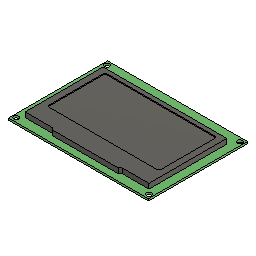
2719 OLED 2.4in (Autodesk Fusion 360 design; units mm, degrees)
Autodesk Fusion 360 part; units mm, degrees
sketch "pcb" plane through (0, 0, 0) normal (0, 0, 1) x (1, 0, 0)
  line L0 (-35, 24.8) -> (35, 24.8)
  line L1 (35, 24.8) -> (35, -24.8)
  line L2 (35, -24.8) -> (-35, -24.8)
  line L3 (-35, -24.8) -> (-35, 24.8)
  line L4 (0, 24.8) -> (0, 0) construction
  line L5 (0, 0) -> (-35, 0) construction
  dimension "d1" = 70
  dimension "d2" = 49.6
  constraint horizontal L0
  constraint vertical L1
  constraint horizontal L2
  constraint vertical L3
  constraint midpoint L0 L4.start
  constraint perpendicular L0 L4
  constraint perpendicular L4 L5
  constraint coincident L4.end L5.start
  constraint midpoint L3 L5.end
  measures "d1" distance of L0.start L0.end
  measures "d2" distance of L0.start L2.end
sketch "holes" plane through (0, 0, 0) normal (0, 0, 1) x (1, 0, 0)
  line L0 (-33.25, 22.75) -> (33.25, 22.75) construction
  line L1 (33.25, 22.75) -> (33.25, -22.75) construction
  line L2 (33.25, -22.75) -> (-33.25, -22.75) construction
  line L3 (-33.25, -22.75) -> (-33.25, 22.75) construction
  line L4 (0, 22.75) -> (0, 0) construction
  line L5 (0, 0) -> (-33.25, 0) construction
  circle A0 centre (-33.25, 22.75) radius 1.25
  circle A1 centre (33.25, 22.75) radius 1.25
  circle A2 centre (33.25, -22.75) radius 1.25
  circle A3 centre (-33.25, -22.75) radius 1.25
  dimension "d3" = 66.5
  dimension "d4" = 45.5
  dimension "d5" = 2.5
  constraint horizontal L0
  constraint vertical L1
  constraint horizontal L2
  constraint vertical L3
  constraint midpoint L0 L4.start
  constraint perpendicular L0 L4
  constraint perpendicular L4 L5
  constraint midpoint L3 L5.end
  constraint coincident L4.end L5.start
  constraint coincident L0.start L3.end
  constraint symmetric L4 A0 A1
  constraint symmetric L5 A0 A3
  constraint symmetric L5 A1 A2
  measures "d3" distance of L0.start L0.end
  measures "d4" distance of L0.start L2.end
  measures "d5" diameter of A0
sketch "bezel" plane through (0, 0, 0) normal (0, 0, 1) x (1, 0, 0)
  line L0 (-31, 18.5) -> (31, 18.5)
  line L1 (31, 18.5) -> (31, -20.5)
  line L2 (31, -20.5) -> (-31, -20.5)
  line L3 (-31, -20.5) -> (-31, 18.5)
  line L4 (0, 18.5) -> (0, -1) construction
  line L5 (0, -1) -> (-31, -1) construction
  line L6 (-17.5, -20.5) -> (-16.5, -21.5)
  line L7 (-16.5, -21.5) -> (16.5, -21.5)
  line L8 (16.5, -21.5) -> (17.5, -20.5)
  line L9 (0, -21.5) -> (0, -20.5) construction
  dimension "d6" = 62
  dimension "d7" = 39
  dimension "d10" = 1
  dimension "d25" = 45
  dimension "d26" = 1
  dimension "d27" = 33
  constraint horizontal L0
  constraint vertical L1
  constraint horizontal L2
  constraint vertical L3
  constraint midpoint L0 L4.start
  constraint perpendicular L0 L4
  constraint perpendicular L4 L5
  constraint midpoint L3 L5.end
  constraint coincident origin L4
  constraint coincident L2 L6.start
  constraint parallel L2 L7
  constraint coincident L2 L8.end
  constraint perpendicular L6 L8
  constraint midpoint L7 L9.start
  constraint perpendicular L7 L9
  constraint midpoint L2 L9.end
  measures "d6" distance of L0.start L0.end
  measures "d7" distance of L0.start L2.end
  measures "d10" distance of origin L5
  measures "d25" angle of L2 L6
  measures "d26" distance of L2 L7
  measures "d27" distance of L6.end L7.end
extrude "Extrude1" add sketch "pcb" along normal blind 1 makes body 1
extrude "Extrude2" cut sketch "holes" along normal blind 1 bodies 1
extrude "Extrude3" add sketch "bezel" along normal blind 2.5 from surface at 1 separate body contours L0 L1 L2 L3 makes body 2
sketch "frame" plane through (0, 0, 3.5) normal (0, 0, 1) x (-1, 0, 0)
  line L0 (31, -18.5) -> (31, 20.5)
  line L1 (31, 20.5) -> (-31, 20.5)
  line L2 (-31, 20.5) -> (-31, -18.5)
  line L3 (-31, -18.5) -> (31, -18.5)
  line L4 (28, -16.5) -> (-28, -16.5)
  line L5 (-28, -16.5) -> (-28, 12.5)
  line L6 (-28, 12.5) -> (28, 12.5)
  line L7 (28, 12.5) -> (28, -16.5)
  line L8 (0, -16.5) -> (0, -2) construction
  line L9 (0, -2) -> (28, -2) construction
  dimension "d18" = 56
  dimension "d19" = 29
  dimension "d20" = 2
  constraint horizontal L4
  constraint vertical L5
  constraint horizontal L6
  constraint vertical L7
  constraint midpoint L4 L8.start
  constraint perpendicular L4 L8
  constraint perpendicular L8 L9
  constraint midpoint L7 L9.end
  constraint coincident origin L8
  measures "d18" distance of L5.end L6.end
  measures "d19" distance of L4.end L5.end
  measures "d20" distance of L3 L4
extrude "Extrude4" cut sketch "frame" against normal blind 0.5 contours L4 L5 L6 L7 bodies 2
fillet "Fillet1" radius 1 4 edges at (-28, 16.5, 3.25) (-28, -12.5, 3.25) (28, 16.5, 3.25) (28, -12.5, 3.25) on bodies 2
extrude "Extrude5" add sketch "bezel" along normal up to surface (2.5 mm away) from surface at 1 contours L2 L6 L7 L8 bodies 2
